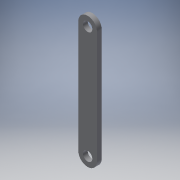
# Autodesk Inventor part: arm4_4
Saved by Autodesk Inventor 2016 (Build 200138000, 138)
## iProperties
Created: 2017-09-18
Part Number: arm4_4
Material: Generic
Document SubType Name: Modeling
Designer: student
Density: 1 g/cm^3
Appearance: Default
Author: student
Autodesk Inventor part; units mm, degrees
ref_plane "YZ Plane" through (0, 0, 0) normal (1, 0, 0) x (0, 1, 0)
ref_plane "XZ Plane" through (0, 0, 0) normal (0, 1, 0) x (-1, 0, 0)
ref_plane "XY Plane" through (0, 0, 0) normal (0, 0, 1) x (1, 0, 0)
sketch "Sketch1" plane through (0, 0, 0) normal (0, 0, 1) x (1, 0, 0)
  line L0 (0, 0) -> (0, 76.2) construction
  line L1 (6.35, 0) -> (6.35, 76.2)
  line L2 (-6.35, 76.2) -> (-6.35, 0)
  arc A0 (-6.35, 0) -> (6.35, 0) centre (0, 0) ccw
  arc A1 (6.35, 76.2) -> (-6.35, 76.2) centre (0, 76.2) ccw
  line L3 (0, 0) -> (76.2, 0) construction
  circle A2 centre (0, 0) radius 3.175
  circle A3 centre (0, 76.2) radius 3.175
  point P0 (0, 38.1)
  dimension "d0" = 76.2
  dimension "d1" = 90
  dimension "d2" = 12.7
  dimension "d3" = 6.35
  dimension "d4" = 6.35
  constraints: 10 end point, 4 centre point, 4 point on circle, 4 tangent, 2 coincident, 1 horizontal, 1 midpoint, 1 parallel, 1 perpendicular, 1 vertical
  measures "d0" distance of L0.start L0.end
  measures "d1" angle of L3 L0
  measures "d2" diameter of A1
  measures "d3" diameter of A2
  measures "d4" diameter of A3
extrude "Extrusion1" add sketch "Sketch1" along normal blind 3.175
body "Solid1"
